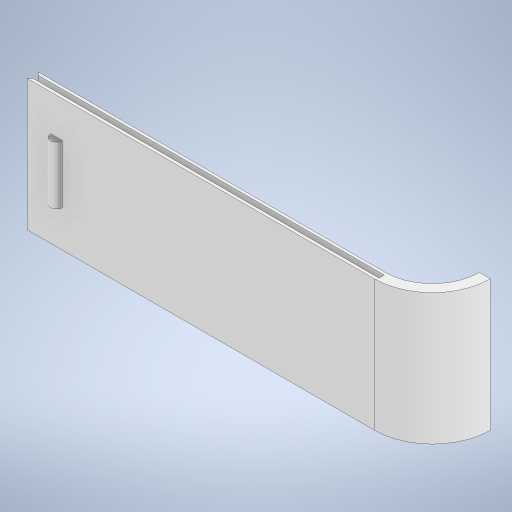
# Autodesk Inventor part: DOOR
Saved by Autodesk Inventor 2023 (Build 270158000, 158)
## iProperties
Created: 2023-03-15
Part Number: DOOR
Material: PC/ABS Plastic
Document SubType Name: Modeling
Designer: Amos Yu
Density: 0.357273 g/cm^3
Appearance: White
Author: Amos Yu
Autodesk Inventor part; units mm, degrees
ref_plane "YZ Plane" through (0, 0, 0) normal (1, 0, 0) x (0, 1, 0)
ref_plane "XZ Plane" through (0, 0, 0) normal (0, 1, 0) x (-1, 0, 0)
sketch "Sketch1" plane through (0, 0, 0) normal (0, 1, 0) x (-1, 0, 0)
  line L0 (0, 0) -> (-59.8, 0)
  arc A0 (-59.8, 0) -> (-69.8, -10) centre (-59.8, -10) ccw
  line L1 (0, -1.9) -> (-59.8, -1.9)
  arc A1 (-59.8, -1.9) -> (-67.9, -10) centre (-59.8, -10) ccw
  line L2 (0, 0) -> (0, -1.9)
  line L3 (-67.9, -10) -> (-69.8, -10)
  dimension "d4" = 10
  dimension "d5" = 69.8
  dimension "d6" = 1.9
  constraints: 8 end point, 4 point on circle, 2 centre point, 1 horizontal, 1 horizontal alignment, 1 perpendicular, 1 tangent, 1 vertical, 1 other
  measures "d4" distance from line of L0 A0.centre
  measures "d5" horizontal distance of L3.end L0.start
  measures "d6" distance between parallel lines of L0 L1
extrude "Extrusion1" add sketch "Sketch1" along normal mid plane 22.6
sketch "Sketch3" plane through (0, 0, 0) normal (1, 0, 0) x (0, 1, 0)
  line L0 (-11.3, -0.5) -> (-8.1, -0.5)
  line L1 (-8.1, -0.5) -> (-8.1, -1.4)
  line L2 (-8.1, -1.4) -> (-11.3, -1.4)
  line L3 (-11.3, -1.4) -> (-11.3, -0.5)
  line L4 (-11.3, 0) -> (-11.3, -1.9) construction
  line L5 (-11.8, -1.9) -> (-7.6, -1.9)
  line L6 (-7.6, -1.9) -> (-7.6, 0)
  line L7 (-7.6, 0) -> (-11.8, 0)
  line L8 (-11.8, 0) -> (-11.8, -1.9)
  point P0 (0, 0)
  point P1 (-11.3, -0.95)
  dimension "d11" = 3.2
  dimension "d12" = 0.9
  dimension "d18" = 0.5
  dimension "d19" = 0.5
  dimension "d20" = 0.5
  dimension "d21" = 0.5
  constraints: 16 end point, 4 parallel, 2 horizontal, 2 midpoint, 2 perpendicular
  measures "d11" distance of L1.end L2.end
  measures "d12" distance of L0.end L1.end
  measures "d18" distance between parallel lines of L1 L6
  measures "d19" distance between parallel lines of L0 L7
  measures "d20" distance between parallel lines of L8 L3
  measures "d21" distance between parallel lines of L5 L2
extrude "Extrusion2" cut sketch "Sketch3" along normal blind 60.1 contours L0 L1 L2 L3
sketch "Sketch3 outline for Extrusion3" plane through (0, 0, 0) normal (1, 0, 0) x (0, 1, 0)
  line L0 (-11.8, -1.9) -> (-7.6, -1.9)
  line L1 (-11.8, 0) -> (-11.8, -1.9)
  line L2 (-7.6, 0) -> (-11.8, 0)
  line L3 (-7.6, -1.9) -> (-7.6, 0)
extrude "Extrusion3" cut sketch "Sketch3 outline for Extrusion3" along normal blind 0.5 draft -45
mirror "Mirror1" about plane through (0, 0, 0) normal (0, 1, 0) of "Extrusion2", "Extrusion3"
ref_plane "Work Plane1" through (0, 0, 0) normal (0, -1, 0) x (1, 0, 0)
sketch "Sketch4" plane through (0, 0, 0) normal (0, -1, 0) x (1, 0, 0)
  line L0 (67.9, -10) -> (69.8, -10)
  arc A0 (69.571144, -10) -> (68.263474, -10) centre (68.917309, -10.25) ccw
  point P0 (0, 0)
  dimension "d26" = 0.7
  dimension "d27" = 0.25
  constraints: 2 point on circle, 2 point on line, 1 centre point
  measures "d26" radius of A0
  measures "d27" distance from line of L0 A0.centre
extrude "Extrusion4" cut sketch "Sketch4" along normal mid plane 10.4
sketch "Sketch5" plane through (0, 0, 0) normal (0, 1, 0) x (-1, 0, 0)
  arc A0 (-4, 0) -> (-6, 0) centre (-5, 0) ccw
  line L0 (-6, 0) -> (-4, 0)
  line L1 (-59.8, 0) -> (0, 0) construction
  dimension "d30" = 1
  dimension "d31" = 5
  constraints: 3 horizontal alignment, 2 end point, 2 point on circle, 1 centre point, 1 collinear
  measures "d30" radius of A0
  measures "d31" distance of A0.centre L1.end
extrude "Extrusion5" add sketch "Sketch5" along normal mid plane 10
equation "\"d4\" = fillet_outer_radius"
equation "\"d5\" = -fillet_outer_radius + total_width - 2 * tol"
equation "\"d6\" = thickness - tol"
equation "\"d7\" = door_height - 4 * tol"
equation "\"d11\" = door_rail_height + 2 * tol"
equation "\"d12\" = door_rail_depth + 4 * tol"
equation "\"d18\" = door_rail_depth"
equation "\"d19\" = door_rail_depth"
equation "\"d20\" = door_rail_depth"
equation "\"d21\" = door_rail_depth"
equation "\"d13\" = -2 * fillet_outer_radius + total_width + tol"
equation "\"d22\" = door_rail_depth"
equation "\"d26\" = door_strike_radius + 2 * tol"
equation "\"d28\" = door_strike_height + 4 * tol"
equation "\"d30\" = door_handle_radius"
equation "\"d31\" = door_handle_inset_width"
equation "\"d32\" = door_handle_height"
equation "\"door_handle_inset_width\" = 5"
equation "\"door_handle_height\" = 10"
equation "\"door_handle_radius\" = 1"
equation "\"fillet_outer_radius\" = 10"
equation "\"total_width\" = 80"
equation "\"tol\" = 0.1"
equation "\"thickness\" = 2"
equation "\"door_height\" = 23"
equation "\"door_rail_height\" = 3"
equation "\"door_rail_depth\" = 0.5"
equation "\"door_strike_radius\" = 0.5"
equation "\"door_strike_height\" = 10"
body "Solid1"
